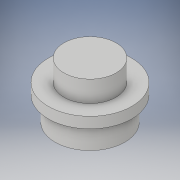
# Autodesk Inventor part: 1x1 circular almost looks like peg peg
Saved by Autodesk Inventor 2017 (Build 210142000, 142)
## iProperties
Created: 2018-05-15
Part Number: 1x1 circular almost looks like peg peg
Material: Generic
Document SubType Name: Modeling
Designer: 20000650
Density: 1 g/cm^3
Appearance: Default
Author: 20000650
Autodesk Inventor part; units mm, degrees
ref_plane "YZ Plane" through (0, 0, 0) normal (1, 0, 0) x (0, 1, 0)
ref_plane "XZ Plane" through (0, 0, 0) normal (0, 1, 0) x (-1, 0, 0)
ref_plane "XY Plane" through (0, 0, 0) normal (0, 0, 1) x (1, 0, 0)
sketch "Sketch1" plane through (0, 0, 0) normal (0, 1, 0) x (-1, 0, 0)
  circle A0 centre (0, 0) radius 2.4498
  circle A1 centre (0, 0) radius 3.2766
  circle A2 centre (0, 0) radius 3.8989
  dimension "d0" = 4.8997
  dimension "d1" = 6.5532
  dimension "d2" = 7.7978
  constraints: 3 centre point, 3 coincident
  measures "d0" diameter of A0
  measures "d1" diameter of A1
  measures "d2" diameter of A2
extrude "Extrusion1" add sketch "Sketch1" along normal blind 1.9837 contours A0
sketch "Sketch2" plane through (0, 0, 0) normal (0, -1, 0) x (1, 0, 0)
  circle A0 centre (0, 0) radius 3.9243
  dimension "d5" = 7.8486
  constraints: 1 centre point, 1 coincident
  measures "d5" diameter of A0
extrude "Extrusion2" add sketch "Sketch2" along normal blind 1.0211
sketch "Sketch3" plane through (0, -1.0211, 0) normal (0, -1, 0) x (1, 0, 0)
  circle A0 centre (0, 0) radius 3.2766
  circle A1 centre (0, 0) radius 2.4511
  dimension "d8" = 6.5532
  dimension "d9" = 4.9022
  constraints: 2 centre point, 2 coincident
  measures "d8" diameter of A0
  measures "d9" diameter of A1
extrude "Extrusion3" add sketch "Sketch3" along normal blind 2.225
body "Solid1"
